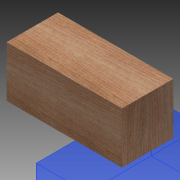
# Autodesk Inventor part: Payload
Saved by Autodesk Inventor 2014 SP2 (Build 180246200, 246)
## iProperties
Created: 2016-04-02
Part Number: Payload
Material: Wood (Birch)
Document SubType Name: Modeling
Designer: hwasserb
Density: 0.480554 g/cm^3
Appearance: Birch - Natural Polished
Mass: 9071.85 g
Surface Area: 4541.93 cm^2
Volume: 18877.9 cm^3
Author: hwasserb
Autodesk Inventor part; units mm, degrees
ref_plane "YZ Plane" through (0, 0, 0) normal (1, 0, 0) x (0, 1, 0)
ref_plane "XZ Plane" through (0, 0, 0) normal (0, 1, 0) x (-1, 0, 0)
ref_plane "XY Plane" through (0, 0, 0) normal (0, 0, 1) x (1, 0, 0)
sketch "Sketch1" plane through (0, 0, 0) normal (1, 0, 0) x (0, 1, 0)
  line L0 (0, 0) -> (203.2, 0)
  line L1 (203.2, 0) -> (203.2, 203.2)
  line L2 (203.2, 203.2) -> (0, 203.2)
  line L3 (0, 203.2) -> (0, 0)
  dimension "d0" = 203.2
  dimension "d1" = 203.2
  constraints: 8 end point, 2 parallel, 1 horizontal, 1 perpendicular
  measures "d0" distance of L2.end L1.end
  measures "d1" distance of L1.end L0.end
extrude "Extrusion1" add sketch "Sketch1" along normal blind 457.2
body "Solid1"
